DHECsensorlid (Autodesk Fusion 360 design; units mm, degrees)
Autodesk Fusion 360 part; units mm, degrees
sketch "Sketch1" plane through (0, 0, 0) normal (0, 1, 0) x (1, 0, 0)
  line L0 (0, 0) -> (35, 0)
  line L1 (35, 0) -> (35, -19)
  line L2 (35, -19) -> (0, -19)
  line L3 (0, -19) -> (0, 0)
  line L4 (0, -19) -> (-0.9, -19)
  line L5 (-0.9, -19) -> (-0.9, -19.9)
  line L6 (-0.9, -19.9) -> (0, -19.9)
  line L7 (0, -19.9) -> (0, -21)
  line L8 (0, -21) -> (35, -21)
  line L9 (35, -21) -> (35, -19.9)
  line L10 (35, -19.9) -> (35.9, -19.9)
  line L11 (35.9, -19.9) -> (35.9, -19)
  line L12 (35.9, -19) -> (35, -19)
  dimension "d2" = 19
  dimension "d3" = 0.9
  dimension "d4" = 0.9
  dimension "d5" = 1.1
  dimension "d17" = 35
  constraint horizontal L0
  constraint vertical L1
  constraint horizontal L2
  constraint vertical L3
  constraint coincident L0.start L3.end
  constraint perpendicular L3 L4
  constraint perpendicular L2 L5
  constraint perpendicular L5 L6
  constraint perpendicular L2 L7
  constraint perpendicular L7 L8
  constraint perpendicular L8 L9
  constraint perpendicular L9 L10
  constraint perpendicular L8 L11
  constraint coincident L2.end L7
  constraint equal L4 L12
  constraint coincident L1.end L9
  constraint coincident L2.end L12
  constraint equal L5 L11
  measures "d2" distance of L0.start L2.end
  measures "d3" distance of L2.end L6
  measures "d4" distance of L5 L7
  measures "d5" distance of L6 L8
  measures "d17" distance of L1 L3
extrude "Extrude1" add sketch "Sketch1" along normal blind 48 contours L2 L4 L5 L6 L7 L8 L9 L10 L11 L12
extrude "Extrude2" add sketch "Sketch1" along normal blind 2 contours L0 L1 L2 L3
sketch "Sketch3" plane through (0, 0, 21) normal (0, 0, 1) x (-1, 0, 0)
  line L0 (0, 0) -> (-35, 0)
  line L1 (-35, 0) -> (-35, -48)
  line L2 (-35, -48) -> (0, -48)
  line L3 (0, -48) -> (0, 0)
  circle A0 centre (-24.25, -37.75) radius 8.25
  circle A1 centre (-24.25, -12.25) radius 8.25
  line L4 (-3, -46) -> (-36, -46) construction
  line L5 (-32.5, -48) -> (-32.5, 0) construction
  line L6 (-36, -4) -> (-3, -4) construction
  circle A2 centre (-5, -37.75) radius 3.75
  dimension "d10" = 16.5
  dimension "d11" = 2
  dimension "d12" = 2.5
  dimension "d13" = 42
  dimension "d14" = 7.5
  dimension "d15" = 5
  constraint equal A0 A1
  constraint vertical A0.centre A1.centre
  constraint perpendicular L1 L4
  constraint tangent A0 L4
  constraint coincident L2 L5.start
  constraint coincident L0 L5.end
  constraint perpendicular L0 L5
  constraint tangent A0 L5
  constraint perpendicular L3 L6
  constraint tangent A1 L6
  constraint horizontal A0.centre A2.centre
  measures "d10" diameter of A0
  measures "d11" distance of L2 L4
  measures "d12" distance of L1 L5
  measures "d13" distance of L4 L6
  measures "d14" diameter of A2 L1
  measures "d15" distance of L3 A2.centre
extrude "Extrude3" cut sketch "Sketch3" against normal through all contours A0 | A1 | A2
